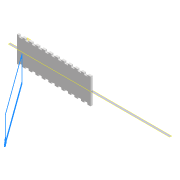
# Autodesk Inventor part: 00_Baseplate_Simmo_side3
Saved by Autodesk Inventor 2022 (Build 260153000, 153)
## iProperties
Created: 2022-04-28
Part Number: 00_Baseplate_Simmo_side3
Material: Generisch
Document SubType Name: Modeling
Designer: diederichbenedict
Density: 1 g/cm^3
Appearance: Vorgabe
Author: diederichbenedict
Autodesk Inventor part; units mm, degrees
ref_plane "YZ Plane" through (0, 0, 0) normal (1, 0, 0) x (0, 1, 0)
ref_plane "XZ Plane" through (0, 0, 0) normal (0, 1, 0) x (-1, 0, 0)
ref_plane "XY Plane" through (0, 0, 0) normal (0, 0, 1) x (1, 0, 0)
ref_plane "Arbeitsebene1" through (0, 0, 0) normal (0, 0, 1) x (1, 0, 0)
sketch "Skizze1" plane through (0, 0, 0) normal (0, 0, 1) x (1, 0, 0)
  line L0 (0, 5) -> (10, 5) projected
  line L1 (10, 0) -> (0, 0) projected
  line L2 (10, 0) -> (10, 5) projected
  line L3 (442.7944, 5) -> (442.7944, 0) projected
  line L4 (0, -68) -> (10, -68) projected
  line L5 (0, 5) -> (230.1, 5)
  line L6 (230.1, 5) -> (230.1, -68)
  line L7 (230.1, -68) -> (0, -68)
  line L8 (0, -68) -> (0, 5)
  line L9 (0, -68) -> (230.1, -68)
  line L10 (230.1, -68) -> (230.1, -74)
  line L11 (230.1, -74) -> (0, -74)
  line L12 (0, -74) -> (0, -68)
  line L13 (0, 0) -> (0, 5) projected
  line L14 (238.603, -69) -> (238.603, -74) projected
  line L15 (230.1, -69) -> (230.1, -74) projected
  line L16 (230.1, -74) -> (220.1, -74) projected
  point P0 (450, -68)
  point P1 (450, 0)
  point P2 (442.7944, 5)
  point P3 (450, -68)
  dimension "d0" = 6
  dimension "d23" = 0
  dimension "d24" = 0
  constraints: 16 end point, 4 parallel, 2 horizontal, 2 perpendicular
  measures "d0" distance of L6.end L10.end
  measures "d23" distance between parallel lines of L15 L10
  measures "d24" distance between parallel lines of L16 L11
extrude "Extrusion1" add sketch "Skizze1" along normal blind 6
sketch "Skizze2" plane through (0, 0, 0) normal (0, 0, -1) x (1, 0, 0)
  line L0 (20, 0) -> (20, -5) projected
  line L1 (10, -5) -> (10, 0) projected
  line L2 (0, -5) -> (0, 74) projected
  line L3 (9.8, -5) -> (20.2, -5)
  line L4 (20.2, -5) -> (20.2, 0)
  line L5 (20.2, 0) -> (9.8, 0)
  line L6 (9.8, 0) -> (9.8, -5)
  point P0 (0, 0)
  dimension "d6" = 0
  dimension "d17" = 0.2
  dimension "d18" = 0.2
  constraints: 8 end point, 2 parallel, 1 horizontal, 1 perpendicular
  measures "d6" distance from line of L1.end L5
  measures "d17" distance between parallel lines of L4 L0
  measures "d18" distance between parallel lines of L6 L1
extrude "Extrusion2" cut sketch "Skizze2" against normal blind 6
sketch "Skizze3" plane through (20.2, 5, 0) normal (0, 1, 0) x (1, 0, 0)
  line L0 (209.9, 0) -> (0, 0) projected
  line L1 (-10.4, -6) -> (0, -6) projected
  line L2 (0, 0) -> (0, -6) projected
  circle A0 centre (-5.2, -3) radius 1.5
  line L3 (-10.4, -6) -> (-10.4, 0) projected
  point P0 (-20.2, 0)
  point P1 (4.8, 3)
  point P2 (429.8, 0)
  point P3 (429.8, -6)
  dimension "d16" = 3
  dimension "d19" = 5.2
  constraints: 1 centre point
  measures "d16" diameter of A0
  measures "d19" distance from line of A0.centre L3
hole "Bohrung1" at (15, 5, 3) direction (0, -1, 0) diameter 3 depth 20
pattern_linear "Rechteckige Anordnung1" count 24 spacing 20 along (1, 0, 0) of "Extrusion2", "Bohrung1"
ref_plane "Arbeitsebene2" through (0, -34.5, 0) normal (0, -1, 0) x (1, 0, 0)
mirror "Spiegeln1" about plane through (0, -34.5, 0) normal (0, -1, 0) of "Extrusion2", "Bohrung1", "Rechteckige Anordnung1"
sketch "Skizze4" plane through (0, 5, 6) normal (0, 1, 0) x (1, 0, 0)
  line L0 (9.8356, 19.8689) -> (14.6897, 16.3421) projected
  line L1 (20.45, 24.2705) -> (14.6897, 16.3421) projected
  line L2 (15.5959, 27.7972) -> (20.45, 24.2705) projected
  line L3 (15.5959, 27.7972) -> (9.8356, 19.8689) projected
  line L4 (9.8, 0) -> (0, 0) projected
  line L5 (3, 0) -> (-2.0103, 0)
  line L6 (-2.0103, 0) -> (-2.0103, 6)
  line L7 (-2.0103, 6) -> (3, 6)
  line L8 (3, 6) -> (3, 0)
  line L9 (0, 6) -> (0, 0) projected
  line L10 (2.8165, 0) -> (2.8165, 6)
  point P0 (-2.0103, 2.2794)
  point P1 (0, 6)
  point P2 (0, 0)
  point P3 (0, 0)
  dimension "d25" = 3
  constraints: 10 end point, 2 parallel, 1 horizontal, 1 perpendicular, 1 point on line, 1 vertical, 3 other
  measures "d25" distance between parallel lines of L9 L8
extrude "Extrusion3" cut sketch "Skizze4" against normal through all contours L3 L2 L1 L0 | L4 L9 L7 L10 | L5 L6 L7 L9
